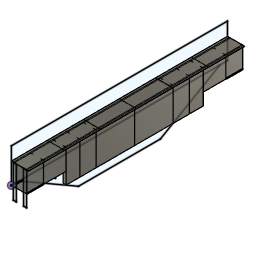
Group 311 Final Bridge (Autodesk Fusion 360 design; units mm, degrees)
Autodesk Fusion 360 part; units mm, degrees
sketch "Design Space" plane through (0, 0, 0) normal (1, 0, 0) x (0, 1, 0)
  line L0 (0, 0) -> (1260, 0)
  line L1 (1260, 0) -> (1260, 200)
  line L2 (1260, 200) -> (0, 200)
  line L3 (0, 200) -> (0, 0)
  line L4 (0, 0) -> (45, 0)
  line L5 (45, 0) -> (391.4102, -200)
  line L6 (391.4102, -200) -> (868.5898, -200)
  line L7 (868.5898, -200) -> (1215, 0)
  dimension "d1" = 1260
  dimension "d2" = 200
  dimension "d4" = 30
  dimension "d5" = 200
  dimension "d6" = 45
  dimension "d7" = 30
  dimension "d68" = 45
  constraint horizontal L0
  constraint vertical L1
  constraint horizontal L2
  constraint vertical L3
  constraint coincident L0.start L3.end
  constraint coincident L0 L4.end
  constraint parallel L0 L6
  constraint coincident L0 L7.end
  measures "d1" distance of L1.end L2.end
  measures "d2" distance of L0.start L2.end
  measures "d4" angle of L0 L5
  measures "d5" distance of L0 L6
  measures "d6" distance of L0.end L7.end
  measures "d7" angle of L0 L7
  measures "d68" distance of L0.start L4.end
sketch "Cross1" plane through (0, 0, 0) normal (0, 1, 0) x (1, 0, 0)
  line L0 (10, 0) -> (90, 0)
  line L1 (90, -1.27) -> (10, -1.27)
  line L2 (10, -1.27) -> (11.27, -1.27)
  line L3 (11.27, -2.54) -> (11.27, -120)
  line L4 (10, -101.27) -> (10, -1.27)
  line L5 (0, -121.27) -> (0, -108)
  line L6 (0, -121.27) -> (100, -121.27)
  line L7 (100, -121.27) -> (100, -122.54)
  line L8 (100, -122.54) -> (0, -122.54)
  line L9 (0, -122.54) -> (0, -121.27)
  line L10 (90, -1.27) -> (88.73, -1.27)
  line L11 (88.73, -2.54) -> (88.73, -120)
  line L12 (88.73, -121.27) -> (90, -121.27)
  line L13 (90, -121.27) -> (90, -1.27)
  line L14 (16.27, -120) -> (16.27, -121.27)
  line L15 (16.27, -120) -> (11.27, -120)
  line L16 (83.73, -120) -> (83.73, -121.27)
  line L17 (83.73, -120) -> (88.73, -120)
  line L18 (0, -122.54) -> (100, -122.54)
  line L19 (100, -122.54) -> (100, -123.81)
  line L20 (100, -123.81) -> (0, -123.81)
  line L21 (0, -123.81) -> (0, -122.54)
  line L22 (90, 0) -> (91.27, 0)
  line L23 (91.27, 0) -> (91.27, -7)
  line L24 (91.27, -7) -> (90, -7)
  line L25 (10, 0) -> (8.73, 0)
  line L26 (8.73, 0) -> (8.73, -7)
  line L27 (8.73, -7) -> (10, -7)
  line L28 (88.73, -2.54) -> (88.73, -1.27)
  line L29 (11.27, -2.54) -> (11.27, -1.27)
  line L30 (10, -101.27) -> (10, -121.27)
  dimension "d24" = 1.27
  dimension "d25" = 1.27
  dimension "d27" = 1.27
  dimension "d28" = 100
  dimension "d29" = 10
  dimension "d30" = 1.27
  dimension "d31" = 5
  dimension "d32" = 1.27
  dimension "d33" = 5
  dimension "d34" = 1.27
  dimension "d37" = 1.27
  dimension "d38" = 100
  dimension "d66" = 120
  dimension "d67" = 80
  dimension "d69" = 1.27
  dimension "d70" = 7
  dimension "d71" = 1.27
  dimension "d72" = 7
  constraint horizontal L0
  constraint horizontal L1
  constraint horizontal L2
  constraint vertical L3
  constraint vertical L4
  constraint horizontal L6
  constraint vertical L7
  constraint horizontal L8
  constraint vertical L9
  constraint horizontal L10
  constraint vertical L11
  constraint horizontal L12
  constraint vertical L13
  constraint coincident L6 L12.start
  constraint coincident L6 L14.end
  constraint perpendicular L6 L14
  constraint perpendicular L3 L15
  constraint coincident L6 L16.end
  constraint perpendicular L6 L16
  constraint perpendicular L11 L17
  constraint horizontal L18
  constraint vertical L19
  constraint horizontal L20
  constraint vertical L21
  constraint perpendicular L0 L23
  constraint coincident L13 L24.end
  constraint perpendicular L13 L24
  constraint perpendicular L25 L26
  constraint coincident L4 L27.end
  constraint perpendicular L4 L27
  constraint perpendicular L10 L28
  constraint perpendicular L2 L29
  constraint coincident L6 L30.end
  constraint perpendicular L6 L30
  measures "d24" distance of L3 L4
  measures "d25" distance of L0 L1
  measures "d27" distance of L6 L8
  measures "d28" distance of L7.end L8.end
  measures "d29" distance of L6.end L12.end
  measures "d30" distance of L11 L13
  measures "d31" distance of L3.end L14.start
  measures "d32" distance of L14.start L14.end
  measures "d33" distance of L11.end L16.start
  measures "d34" distance of L16.start L16.end
  measures "d37" distance of L18 L20
  measures "d38" distance of L19.end L20.end
  measures "d66" distance of L1.start L12.end
  measures "d67" distance of L0.start L0.end
  measures "d69" distance of L4 L26
  measures "d70" distance of L25 L27
  measures "d71" distance of L13 L23
  measures "d72" distance of L22.end L23.end
extrude "Extrude9" add sketch "Cross1" along normal blind 420 contours L8 L18 L19 L20 L21 makes body 1
extrude "Extrude10" add sketch "Cross1" along normal blind 420 from surface at 420 separate body contours L8 L18 L19 L20 L21 makes body 2
extrude "Extrude11" add sketch "Cross1" along normal blind 420 separate body contours L8 L18 L19 L20 L21 makes body 3
move_face "MoveFace1" by (0, 8400, 0) 1 faces at (66.6667, 140, 123.81) on bodies 3
move_face "MoveFace2" by (0, 840, 0) 1 faces at (66.6667, 140, 123.81) on bodies 3
move_body "Move5" bodies 3 to x (1, 0, 0) y (0, 1, 0) z (0, 0, 1) at (0, 840, 0)
extrude "Extrude12" add sketch "Cross1" along normal blind 210 separate body contours L6 L7 L8 L9 L12 L18 makes body 4
extrude "Extrude13" add sketch "Cross1" along normal blind 210 from surface at 1050 separate body contours L6 L7 L8 L9 L12 L18 makes body 5
extrude "Extrude14" add sketch "Cross1" along normal blind 420 from surface at 210 separate body contours L6 L7 L8 L9 L12 L18 makes body 6
extrude "Extrude15" add sketch "Cross1" along normal blind 420 from surface at 210 separate body contours L6 L7 L8 L9 L12 L18 makes body 7
move_body "Move6" bodies 7 to x (1, 0, 0) y (0, 1, 0) z (0, 0, 1) at (0, 420, 0)
extrude "Extrude16" add sketch "Cross1" along normal blind 230 separate body contours L1 L2 L3 L4 L6 L14 L15 L29 L30 | L1 L6 L10 L11 L12 L13 L16 L17 L28 makes body 8 at (90, 153.3333, 81.27) makes body 9 at (10, 76.6667, 81.27)
extrude "Extrude17" add sketch "Cross1" along normal blind 230 from surface at 1030 separate body contours L1 L2 L3 L4 L6 L14 L15 L29 L30 | L1 L6 L10 L11 L12 L13 L16 L17 L28 makes body 10 at (10, 1106.6667, 81.27) makes body 11 at (90, 1183.3333, 81.27)
extrude "Extrude18" add sketch "Cross1" along normal blind 99 separate body contours L0 L1 L2 L4 L10 L13 L22 L23 L24 L25 L26 L27 makes body 12
extrude "Extrude19" add sketch "Cross1" along normal blind 99 from surface at 1161 separate body contours L0 L1 L2 L4 L10 L13 L22 L23 L24 L25 L26 L27 makes body 13
sketch "Sketch13" plane through (0, 0, 0) normal (0, 1, 0) x (1, 0, 0)
  line L0 (10, -121.27) -> (11.27, -121.27)
  line L1 (11.27, -120) -> (11.27, 68.73)
  line L2 (11.27, 68.73) -> (10, 68.73)
  line L3 (10, 68.73) -> (10, -121.27)
  line L4 (10, -101.27) -> (10, -121.27)
  line L5 (88.73, -121.27) -> (90, -121.27)
  line L6 (90, -121.27) -> (90, 68.73)
  line L7 (90, 68.73) -> (88.73, 68.73)
  line L8 (88.73, 68.73) -> (88.73, -120)
  line L9 (90, -121.27) -> (90, -1.27)
  line L10 (11.27, -121.27) -> (16.27, -121.27)
  line L11 (16.27, -121.27) -> (16.27, -120)
  line L12 (16.27, -120) -> (11.27, -120)
  line L13 (88.73, -121.27) -> (83.73, -121.27)
  line L14 (83.73, -121.27) -> (83.73, -120)
  line L15 (83.73, -120) -> (88.73, -120)
  point P0 (0, -121.27)
  dimension "d104" = 190
  dimension "d105" = 1.27
  dimension "d106" = 1.27
  dimension "d107" = 1.27
  dimension "d108" = 190
  dimension "d109" = 1.27
  dimension "d110" = 5
  dimension "d111" = 5
  dimension "d112" = 1.27
  constraint horizontal L0
  constraint vertical L1
  constraint horizontal L2
  constraint vertical L3
  constraint horizontal L0.start P0
  constraint horizontal L5
  constraint vertical L6
  constraint horizontal L7
  constraint vertical L8
  constraint coincident L5.end L6.start
  constraint horizontal L10
  constraint vertical L11
  constraint horizontal L12
  constraint horizontal L13
  constraint vertical L14
  constraint horizontal L15
  measures "d104" distance of L0.start L2.end
  measures "d105" distance of L1 L4
  measures "d106" distance of L1 L3
  measures "d107" distance of L8 L9
  measures "d108" distance of L5.end L6.end
  measures "d109" distance of L10 L12
  measures "d110" distance of L1 L11
  measures "d111" distance of L5.start L13.end
  measures "d112" distance of L13 L15
extrude "Extrude20" add sketch "Sketch13" along normal blind 800 from surface at 230 separate body makes body 14 at (90, 496.6667, 57.9367) makes body 15 at (10, 496.6667, -5.3967)
sketch "Sketch14" plane through (0, 0, 0) normal (0, 1, 0) x (1, 0, 0)
  line L0 (11.27, -121.2469) -> (28.77, -121.2469)
  line L1 (28.77, -121.2469) -> (28.77, -1.2469)
  line L2 (28.77, -1.2469) -> (11.27, -1.2469)
  line L3 (11.27, -1.2469) -> (11.27, -121.2469)
  line L4 (11.27, -2.54) -> (11.27, -120)
  line L5 (88.73, -121.2892) -> (71.23, -121.2892)
  line L6 (71.23, -121.2892) -> (71.23, -1.2892)
  line L7 (71.23, -1.2892) -> (88.73, -1.2892)
  line L8 (88.73, -1.2892) -> (88.73, -121.2892)
  point P0 (88.73, -120)
  dimension "d116" = 120
  dimension "d117" = 17.5
  dimension "d118" = 120
  dimension "d119" = 17.5
  constraint horizontal L0
  constraint vertical L1
  constraint horizontal L2
  constraint vertical L3
  constraint coincident L3 L4.end
  constraint horizontal L5
  constraint vertical L6
  constraint horizontal L7
  constraint vertical L8
  constraint coincident L8 P0
  measures "d116" distance of L0.end L1.end
  measures "d117" distance of L1 L4
  measures "d118" distance of L5.end L6.end
  measures "d119" distance of L6 L8
extrude "Extrude21" add sketch "Sketch14" along normal blind 1.27 separate body makes body 16 at (17.1033, 0, 41.2469) makes body 17 at (82.8967, 0, 81.2892)
extrude "Extrude22" add sketch "Sketch14" along normal blind 1.27 from surface at 1258.73 separate body makes body 18 at (17.1033, 1258.73, 41.2469) makes body 19 at (82.8967, 1258.73, 81.2892)
extrude "Extrude23" add sketch "Sketch14" along normal blind 1.27 from surface at 100 separate body makes body 20 at (17.1033, 100, 41.2469) makes body 21 at (82.8967, 100, 81.2892)
extrude "Extrude24" add sketch "Sketch14" along normal blind 1.27 from surface at 1160 separate body makes body 22 at (17.1033, 1160, 41.2469) makes body 23 at (82.8967, 1160, 81.2892)
extrude "Extrude25" add sketch "Sketch14" along normal blind 1.27 from surface at 228.73 separate body makes body 24 at (17.1033, 228.73, 41.2469) makes body 25 at (82.8967, 228.73, 81.2892)
extrude "Extrude26" add sketch "Sketch14" along normal blind 1.27 from surface at 1028.73 separate body makes body 26 at (17.1033, 1028.73, 41.2469) makes body 27 at (82.8967, 1028.73, 81.2892)
move_body "Move7" bodies 26 27 to x (1, 0, 0) y (0, 1, 0) z (0, 0, 1) at (0, 1.27, 0)
sketch "Sketch15" plane through (0, 0, 0) normal (0, 1, 0) x (1, 0, 0)
  line L0 (11.27, -121.2469) -> (28.77, -121.2469)
  line L1 (28.77, -121.2469) -> (28.77, 68.7531)
  line L2 (28.77, 68.7531) -> (11.27, 68.7531)
  line L3 (11.27, 68.7531) -> (11.27, -121.2469)
  line L4 (71.23, -121.2892) -> (88.73, -121.2892)
  line L5 (88.73, -121.2892) -> (88.73, 68.7108)
  line L6 (88.73, 68.7108) -> (71.23, 68.7108)
  line L7 (71.23, 68.7108) -> (71.23, -121.2892)
  line L8 (11.27, -1.2469) -> (11.27, -121.2469)
  line L9 (71.23, -121.2892) -> (71.23, -1.2892)
  line L10 (88.73, -121.2892) -> (71.23, -121.2892)
  line L11 (11.27, -121.2469) -> (28.77, -121.2469)
  point P0 (11.27, -121.2469)
  point P1 (71.23, -121.2892)
  dimension "d137" = 17.5
  dimension "d138" = 17.5
  dimension "d139" = 190
  dimension "d140" = 190
  constraint horizontal L0
  constraint vertical L1
  constraint horizontal L2
  constraint vertical L3
  constraint horizontal L4
  constraint vertical L5
  constraint horizontal L6
  constraint vertical L7
  constraint coincident P0 L0.start
  constraint coincident P1 L4.start
  measures "d137" distance of L1 L8
  measures "d138" distance of L5 L9
  measures "d139" distance of L6 L10
  measures "d140" distance of L2 L11
extrude "Extrude27" add sketch "Sketch15" along normal blind 1.27 from surface at 230 separate body makes body 28 at (17.1033, 230, -5.4198) makes body 29 at (77.0633, 230, -5.3775)
extrude "Extrude28" add sketch "Sketch15" along normal blind 1.27 from surface at 1028.73 separate body makes body 30 at (17.1033, 1028.73, -5.4198) makes body 31 at (77.0633, 1028.73, -5.3775)
extrude "Extrude29" add sketch "Sketch15" along normal blind 1.27 from surface at 310 separate body makes body 32 at (17.1033, 310, -5.4198) makes body 33 at (77.0633, 310, -5.3775)
extrude "Extrude30" add sketch "Sketch15" along normal blind 1.27 from surface at 948.73 separate body makes body 34 at (17.1033, 948.73, -5.4198) makes body 35 at (77.0633, 948.73, -5.3775)
extrude "Extrude31" add sketch "Sketch15" along normal blind 1.27 from surface at 405 separate body makes body 36 at (17.1033, 405, -5.4198) makes body 37 at (77.0633, 405, -5.3775)
extrude "Extrude32" add sketch "Sketch15" along normal blind 1.27 from surface at 853.73 separate body makes body 38 at (17.1033, 853.73, -5.4198) makes body 39 at (77.0633, 853.73, -5.3775)
extrude "Extrude33" add sketch "Sketch15" along normal blind 1.27 from surface at 629.365 separate body makes body 40 at (17.1033, 629.365, -5.4198) makes body 41 at (77.0633, 629.365, -5.3775)
move_body "Move8" bodies 21 to x (1, 0, 0) y (0, 1, 0) z (0, 0, 1) at (0, -2.27, 0)
move_body "Move9" bodies 20 to x (1, 0, 0) y (0, 1, 0) z (0, 0, 1) at (0, -2.27, 0)
move_body "Move10" bodies 23 to x (1, 0, 0) y (0, 1, 0) z (0, 0, 1) at (0, 1, 0)
move_body "Move11" bodies 22 to x (1, 0, 0) y (0, 1, 0) z (0, 0, 1) at (0, 1, 0)
move_body "Move12" bodies 21 to x (1, 0, 0) y (0, 1, 0) z (0, 0, 1) at (0, 0.33, 0)
move_body "Move13" bodies 21 to x (1, 0, 0) y (0, 1, 0) z (0, 0, 1) at (0, -0.06, 0)
move_body "Move14" bodies 21 to x (1, 0, 0) y (0, 1, 0) z (0, 0, 1) at (0, -0.27, 0)
sketch "cross section1" plane through (0, 0, 0) normal (0, 1, 0) x (1, 0, 0)
  line L0 (-10.2399, -76.27) -> (89.7601, -76.27)
  line L1 (89.7601, -76.27) -> (89.7601, -75)
  line L2 (89.7601, -75) -> (-10.2399, -75)
  line L3 (-10.2399, -75) -> (-10.2399, -76.27)
  line L4 (0, -1.27) -> (80, -1.27)
  line L5 (80, -1.27) -> (80, 0)
  line L6 (80, 0) -> (0, 0)
  line L7 (0, 0) -> (0, -1.27)
  line L8 (0, -1.27) -> (1.27, -1.27)
  line L9 (1.27, -1.27) -> (1.27, -75)
  line L10 (1.27, -75) -> (0, -75)
  line L11 (0, -75) -> (0, -1.27)
  line L12 (80, -1.27) -> (78.73, -1.27)
  line L13 (78.73, -1.27) -> (78.73, -75)
  line L14 (78.73, -75) -> (80, -75)
  line L15 (80, -75) -> (80, -1.27)
  dimension "d9" = 1.27
  dimension "d10" = 80
  dimension "d11" = 1.27
  dimension "d13" = 1.27
  dimension "d14" = 1.27
  constraint horizontal L0
  constraint vertical L1
  constraint horizontal L2
  constraint vertical L3
  constraint horizontal L4
  constraint vertical L5
  constraint horizontal L6
  constraint vertical L7
  constraint horizontal L8
  constraint vertical L9
  constraint horizontal L10
  constraint vertical L11
  constraint coincident L2 L9.end
  constraint horizontal L12
  constraint vertical L13
  constraint horizontal L14
  constraint vertical L15
  constraint coincident L2 L13.end
  constraint coincident L6.end L7.start
  measures "d9" distance of L0.end L1.end
  measures "d10" distance of L4.start L4.end
  measures "d11" distance of L4.end L5.end
  measures "d13" distance of L9 L11
  measures "d14" distance of L13 L15
extrude "Extrude1" [suppressed]
sketch "Sketch3" plane through (0, 0, 0) normal (0, 1, 0) x (1, 0, 0)
  line L0 (0, 0) -> (100, 0)
  line L1 (100, 0) -> (100, -200)
  line L2 (100, -200) -> (0, -200)
  line L3 (0, -200) -> (0, 0)
  line L4 (0, 0) -> (100, 0)
  line L5 (100, 0) -> (100, 200)
  line L6 (100, 200) -> (0, 200)
  line L7 (0, 200) -> (0, 0)
  dimension "d17" = 200
  dimension "d18" = 100
  dimension "d19" = 200
  dimension "d20" = 100
  constraint horizontal L0
  constraint vertical L1
  constraint horizontal L2
  constraint vertical L3
  constraint coincident L0.start L3.end
  constraint horizontal L4
  constraint vertical L5
  constraint horizontal L6
  constraint vertical L7
  measures "d17" distance of L0.end L1.end
  measures "d18" distance of L0.start L0.end
  measures "d19" distance of L0.end L5.end
  measures "d20" distance of L5.end L6.end
sketch "Sketch4" plane through (0, 0, 0) normal (0, 1, 0) x (1, 0, 0)
equation "d122 = 1260 mm - 1.27 mm"
equation "d128 = 1260 mm - 100 mm"
equation "d131 = 230 mm - 1.27 mm"
equation "d144 = 1260 mm - 230 mm - 1.27 mm"
equation "d147 = 230 mm + 80 mm"
equation "d150 = 1260 mm - ( 230 mm + 80 mm ) - 1.27 mm"
equation "d156 = 1260 mm - 405 mm - 1.27 mm"
